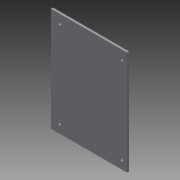
# Autodesk Inventor part: top panel
Saved by Autodesk Inventor 2014 (Build 180170000, 170)
## iProperties
Created: 2014-11-30
Part Number: top panel
Material: Generic
Document SubType Name: Modeling
Designer: ph1140784
Density: 1 g/cm^3
Appearance: Default
Author: ph1140784
Autodesk Inventor part; units mm, degrees
ref_plane "YZ Plane" through (0, 0, 0) normal (1, 0, 0) x (0, 1, 0)
ref_plane "XZ Plane" through (0, 0, 0) normal (0, 1, 0) x (-1, 0, 0)
ref_plane "XY Plane" through (0, 0, 0) normal (0, 0, 1) x (1, 0, 0)
ref_plane "Work Plane1" through (0, 3, 0) normal (0, 1, 0) x (1, 0, 0)
sketch "Sketch2" plane through (0, 3, 0) normal (0, 1, 0) x (1, 0, 0)
  line L0 (-55, -65) -> (55, -65) projected
  line L1 (55, -65) -> (55, 65) projected
  line L2 (-55, 65) -> (-55, -65) projected
  circle A0 centre (47, 72.5) radius 2.5
  circle A1 centre (47, -52.5) radius 2.5
  circle A2 centre (-43, -52.5) radius 2.5
  circle A3 centre (-43, 72.5) radius 2.5
  line L3 (-55, -65) -> (-55, 85)
  line L4 (-55, -65) -> (55, -65)
  line L5 (55, -65) -> (55, 85)
  line L6 (55, 85) -> (-55, 85)
  point P0 (0, 0)
  constraints: 8 end point, 4 centre point, 2 perpendicular, 1 parallel
extrude "Extrusion2" add sketch "Sketch2" along normal blind 3
body "Solid2"
